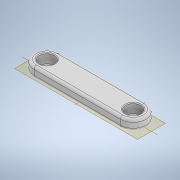
# Autodesk Inventor part: рычаг-1
Saved by Autodesk Inventor 2020.3 (Build 243373000, 373)
## iProperties
Created: 2020-08-24
Part Number: рычаг-1
Material: Типовые
Document SubType Name: Modeling
Designer: Alkhimov
Density: 1 g/cm^3
Appearance: По умолчанию
Author: Alkhimov
Autodesk Inventor part; units mm, degrees
ref_plane "YZ Plane" through (0, 0, 0) normal (1, 0, 0) x (0, 1, 0)
ref_plane "XY Plane" through (0, 0, 0) normal (0, 0, 1) x (1, 0, 0)
sketch "Эскиз1" plane through (0, 0, 0) normal (0, 1, 0) x (-1, 0, 0)
  line L0 (17, 0) -> (-17, 0) construction
  line L1 (17, 5) -> (-17, 5)
  line L2 (-17, -5) -> (17, -5)
  arc A0 (17, -5) -> (17, 5) centre (17, 0) ccw
  arc A1 (-17, 5) -> (-17, -5) centre (-17, 0) ccw
  circle A2 centre (17, 0) radius 3
  circle A3 centre (-17, 0) radius 3
  point P0 (0, 0)
  point P1 (0, 0)
  dimension "d0" = 34
  dimension "d1" = 10
  dimension "d2" = 6
  constraints: 8 end point, 4 centre point, 4 point on circle, 4 tangent, 3 coincident, 1 equal radius, 1 horizontal, 1 midpoint, 1 parallel
  measures "d0" distance of L0.start L0.end
  measures "d1" diameter of A1
  measures "d2" diameter of A2
extrude "Выдавливание1" add sketch "Эскиз1" along normal blind 4
fillet "Сопряжение1" radius 1 8 edges at (22, 4, 0) (0, 4, -5) (-22, 4, 0) (0, 4, 5) (22, 0, 0) (0, 0, -5) (-22, 0, 0) (0, 0, 5)
fillet "Сопряжение2" radius 0.3 4 edges at (-14, 0, 0) (-14, 4, 0) (20, 0, 0) (20, 4, 0)
